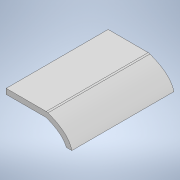
# Autodesk Inventor part: obudowa_czołg
Saved by Autodesk Inventor 2021 (Build 250183000, 183)
## iProperties
Created: 2022-02-09
Part Number: obudowa_czołg
Material: Generic
Document SubType Name: Modeling
Designer: Łukasz
Density: 1 g/cm^3
Appearance: Default
Author: Łukasz
Autodesk Inventor part; units mm, degrees
ref_plane "YZ Plane" through (0, 0, 0) normal (1, 0, 0) x (0, 1, 0)
ref_plane "XZ Plane" through (0, 0, 0) normal (0, 1, 0) x (-1, 0, 0)
ref_plane "XY Plane" through (0, 0, 0) normal (0, 0, 1) x (1, 0, 0)
sketch "Sketch1" plane through (0, 0, 0) normal (0, 0, 1) x (1, 0, 0)
  line L0 (327.1957, 60) -> (246.3077, 60)
  arc A0 (376.3077, 20) -> (352.3671, 47.7862) centre (325, 0) ccw construction
  line L1 (328.3961, 60) -> (328.3961, 20) construction
  line L2 (328.3961, 20) -> (376.3077, 20) construction
  line L3 (376.3077, 20) -> (328.3961, 20) construction
  line L4 (376.3077, 20) -> (506.3077, 20) construction
  line L5 (246.3077, 20) -> (246.3077, 60) construction
  arc A1 (329.4656, 59.455) -> (327.1957, 60) centre (327.1957, 55) ccw
  line L6 (246.3077, 62.5) -> (327.1957, 62.5)
  arc A2 (330.6006, 61.6825) -> (327.1957, 62.5) centre (327.1957, 55) ccw
  line L7 (246.3077, 60) -> (246.3077, 62.5)
  line L8 (376.3077, 20) -> (378.9821, 20)
  spline S0 degree 2 poles (329.4656, 59.455) (368.4042, 45.6401) (376.3077, 20) knots 0 0 0 1 1 1
  line L9 (373.1943, 30.1003) -> (379.421, 9.8997) construction
  arc A3 (377.9878, 11.8329) -> (373.0981, 27.6957) centre (334.7924, 7.2031) ccw construction
  spline S1 degree 2 poles (330.6006, 61.6825) (372.8896, 46.3324) (378.9821, 20) knots 0 0 0 1 1 1
  line L10 (376.7474, 29.6587) -> (381.2168, 10.3413) construction
  arc A4 (379.966, 12.2527) -> (376.4632, 27.3922) centre (341.2659, 11.2737) ccw construction
  point P0 (0, 0)
  point P1 (334.4465, 56.9171)
  dimension "d0" = 40
  dimension "d1" = 130
  dimension "d2" = 180
  dimension "d3" = 5
  dimension "d4" = 2.5
  constraints: 22 end point, 9 point on circle, 5 centre point, 4 midpoint, 3 perpendicular, 2 point on line, 1 collinear, 1 horizontal, 1 tangent, 1 vertical, 8 other
  measures "d0" distance of L1.end L1.start
  measures "d1" distance of L2.end L5.start
  measures "d2" angle of L4 L3
  measures "d3" radius of A1
  measures "d4" distance between parallel lines of L0 L6
extrude "Extrusion1" add sketch "Sketch1" along normal blind 200
sketch "Sketch2" plane through (0, 0, 200) normal (0, 0, 1) x (1, 0, 0)
  spline S0 degree 2 poles (378.9821, 20) (372.8896, 46.3324) (330.6006, 61.6825) knots 0 0 0 1 1 1 projected
  arc A0 (330.6006, 61.6825) -> (327.1957, 62.5) centre (327.1957, 55) ccw projected
  line L0 (327.1957, 62.5) -> (246.3077, 62.5) projected
  spline S1 degree 2 poles (329.4656, 59.455) (368.4042, 45.6401) (376.3077, 20) knots 0 0 0 1 1 1
  line L1 (378.9821, 20) -> (367.844, 20)
  line L2 (326.7907, 51.9155) -> (246.3077, 51.9155)
  line L3 (326.7907, 51.9155) -> (407.2737, 51.9155) construction
  line L4 (246.3077, 51.9155) -> (246.3077, 62.5)
  line L5 (246.3077, 60) -> (327.1957, 60) projected
  spline S2 degree 5 poles (326.7907, 51.9155) (331.1594, 50.3654) (335.4692, 48.6475) (339.6974, 46.7324) (347.0129, 42.9121) (353.7535, 38.1655) (356.5541, 35.8919) (361.3163, 31.2934) (365.1183, 25.8881) (366.6006, 23.2657) (367.7818, 20.5001) (368.6626, 17.6434) knots 0 0 0 0 0 0 0.413162 0.413162 0.413162 0.733543 0.733543 0.733543 1 1 1 1 1 1
  point P0 (0, 0)
  dimension "d7" = 8
  dimension "d8" = 180
  constraints: 8 end point, 2 horizontal, 1 collinear, 1 perpendicular, 6 other
  measures "d8" angle of L2 L3
extrude "Extrusion2" add sketch "Sketch2" along normal blind 3
sketch "Sketch3" plane through (0, 0, 0) normal (0, 0, -1) x (-1, 0, 0)
  line L0 (-246.3077, 60) -> (-327.1957, 60) projected
  arc A0 (-327.1957, 60) -> (-329.4656, 59.455) centre (-327.1957, 55) ccw projected
  line L1 (-367.844, 20) -> (-376.3077, 20) projected
  spline S0 degree 5 poles (-326.7907, 51.9155) (-331.1594, 50.3654) (-335.4692, 48.6475) (-339.6974, 46.7324) (-347.0129, 42.9121) (-353.7535, 38.1655) (-356.5541, 35.8919) (-360.9554, 31.6419) (-364.5365, 26.7029) (-365.8382, 24.5649) (-366.9439, 22.3223) (-367.844, 20) knots 0 0 0 0 0 0 0.432394 0.432394 0.432394 0.767689 0.767689 0.767689 1 1 1 1 1 1 projected
  line L2 (-246.3077, 51.9155) -> (-326.7907, 51.9155) projected
  line L3 (-246.3077, 60) -> (-246.3077, 51.9155) projected
  line L4 (-246.3077, 62.5) -> (-246.3077, 51.9155) projected
  line L5 (-246.3077, 51.9155) -> (-326.7907, 51.9155) projected
  line L6 (-367.844, 20) -> (-378.9821, 20) projected
  spline S1 degree 2 poles (-378.9821, 20) (-372.8896, 46.3324) (-330.6006, 61.6825) knots 0 0 0 1 1 1 projected
  arc A1 (-327.1957, 62.5) -> (-330.6006, 61.6825) centre (-327.1957, 55) ccw projected
  line L7 (-327.1957, 62.5) -> (-246.3077, 62.5) projected
  point P0 (0, 0)
  constraints: 4 other
extrude "Extrusion3" add sketch "Sketch3" along normal blind 3
fillet "Fillet1" radius 4 2 edges at (326.7907, 51.9155, 201.5) (326.7907, 51.9155, -1.5)
body "Solid1"
